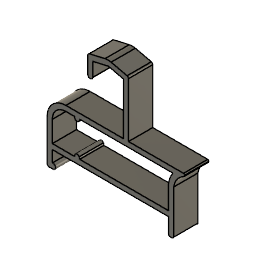
AdaptadorRiel (Autodesk Fusion 360 design; units mm, degrees)
part number: 2025-12-28-18-35-44-628
Autodesk Fusion 360 part; units mm, degrees
sketch "Boceto1" plane through (0, 0, 0) normal (0, 1, 0) x (1, 0, 0)
  line L0 (52.1, -0.6) -> (52.1, -18.5)
  line L1 (0, -17.65) -> (0, -0.6)
  line L2 (2.15, 0) -> (2.7296, 0)
  line L3 (49.95, -0.6) -> (49.95, -6.85)
  line L4 (49.95, -6.85) -> (2.15, -6.85)
  line L5 (2.15, -6.85) -> (2.15, -2.1)
  arc A0 (2.15, -2.1) -> (2.7296, 0) centre (2.4398, -1.05) ccw
  line L6 (0.6, 0) -> (2.7296, 0)
  line L7 (50.55, 0) -> (51.5, 0)
  arc A1 (0.6, 0) -> (0, -0.6) centre (0.6, -0.6) ccw
  arc A2 (50.55, 0) -> (49.95, -0.6) centre (50.55, -0.6) ccw
  arc A3 (52.1, -0.6) -> (51.5, 0) centre (51.5, -0.6) ccw
  arc A4 (0, -17.65) -> (7.75, -25.4) centre (7.75, -17.65) ccw
  line L8 (52.1, -25.4) -> (56.15, -25.4)
  line L9 (56.6, -24.95) -> (56.6, -24.7835)
  arc A5 (52.1, -18.5) -> (56.3513, -24.381) centre (59.8591, -17.3682) ccw
  arc A6 (56.15, -25.4) -> (56.6, -24.95) centre (56.15, -24.95) ccw
  arc A7 (56.6, -24.7835) -> (56.3513, -24.381) centre (56.15, -24.7835) ccw
  line L10 (2.15, -17.65) -> (2.15, -9)
  arc A8 (2.15, -17.65) -> (7.75, -23.25) centre (7.75, -17.65) ccw
  arc A9 (49.95, -18.6465) -> (51.6168, -23.0152) centre (59.8591, -17.3682) ccw
  line L11 (49.95, -9) -> (49.95, -18.6465)
  arc A10 (51.4931, -23.25) -> (51.6168, -23.0152) centre (51.4931, -23.1) ccw
  arc A11 (11.3, -9) -> (11.4993, -9.8229) centre (13.208, -8.9734) ccw
  line L12 (11.4993, -9.8229) -> (13.208, -9.8229) construction
  arc A12 (13.208, -9.8229) -> (13.4, -9) centre (11.5634, -9.0053) ccw
  arc A13 (11.4993, -9.8229) -> (13.208, -9.8229) centre (12.3537, -9.3982) ccw
  line L13 (49.95, -9) -> (13.4, -9)
  line L14 (11.3, -9) -> (2.15, -9)
  arc A14 (11.6218, -22.29) -> (11.3, -23.25) centre (12.6842, -23.18) ccw
  arc A15 (13.4, -23.25) -> (13.0782, -22.29) centre (12.0158, -23.18) ccw
  arc A16 (13.0782, -22.29) -> (11.6218, -22.29) centre (12.35, -22.9) ccw
  line L15 (51.4931, -23.25) -> (13.4, -23.25)
  line L16 (11.3, -23.25) -> (7.75, -23.25)
  line L17 (31.4, -25.4) -> (31.4, -46.6)
  line L18 (31.4, -46.6) -> (25.2, -48.1)
  line L19 (25.2, -48.1) -> (18.8, -46.6231)
  line L20 (18.8, -46.6231) -> (18.8, -40.9)
  line L21 (17.8, -39.9) -> (17.7, -39.9)
  line L22 (16.7, -40.9) -> (16.7, -47.8649)
  arc A17 (18.8, -40.9) -> (17.8, -39.9) centre (17.8, -40.9) ccw
  arc A18 (17.7, -39.9) -> (16.7, -40.9) centre (17.7, -40.9) ccw
  line L23 (23.8484, -50.1112) -> (17.2814, -48.5957)
  line L24 (26.3501, -50.1046) -> (32.9225, -48.5513)
  line L25 (33.5, -47.8214) -> (33.5, -25.4)
  line L26 (52.1, -25.4) -> (33.5, -25.4)
  line L27 (31.4, -25.4) -> (7.75, -25.4)
  arc A19 (16.7, -47.8649) -> (17.2814, -48.5957) centre (17.45, -47.8649) ccw
  arc A20 (32.9225, -48.5513) -> (33.5, -47.8214) centre (32.75, -47.8214) ccw
  arc A21 (23.8484, -50.1112) -> (26.3501, -50.1046) centre (25.0851, -44.752) ccw
  dimension "d1" = 0.6
  dimension "d2" = 7.75
  dimension "d3" = 0.45
  dimension "d5" = 0.15
  dimension "d6" = 1
  dimension "d7" = 0.75
  dimension "d8" = 5.5
  constraint horizontal L6
  constraint vertical L0
  constraint horizontal L26
  constraint vertical L1
  constraint horizontal L2
  constraint vertical L3
  constraint horizontal L4
  constraint vertical L5
  constraint coincident L2.start L6
  constraint collinear L6 L7
  constraint tangent L1 A1
  constraint tangent L6 A1
  constraint tangent L3 A2
  constraint tangent L7 A2
  constraint equal A1 A2
  constraint tangent L0 A3
  constraint tangent L7 A3
  constraint equal A1 A3
  constraint tangent A4 L26
  constraint tangent L1 A4
  constraint perpendicular L0 L8
  constraint perpendicular L8 L9
  constraint tangent L8 A6
  constraint tangent L9 A6
  constraint tangent L9 A7
  constraint tangent A5 A7
  constraint equal A6 A7
  constraint concentric A4 A8
  constraint concentric A5 A9
  constraint tangent L10 A8
  constraint tangent A8 L15
  constraint tangent A10 L15
  constraint tangent A9 A10
  constraint tangent A11 A13
  constraint coincident A11.start L13
  constraint horizontal L12
  constraint collinear L13 L14
  constraint tangent A14 A16
  constraint coincident A14.end L15
  constraint tangent A15 A16
  constraint collinear L15 L16
  constraint coincident L17.start L26
  constraint perpendicular L17 L26
  constraint vertical L20
  constraint perpendicular L20 L21
  constraint perpendicular L21 L22
  constraint tangent L20 A17
  constraint tangent L21 A17
  constraint tangent L21 A18
  constraint tangent L22 A18
  constraint equal A17 A18
  constraint parallel L19 L23
  constraint perpendicular L25 L26
  constraint collinear L26 L27
  constraint tangent L23 A19
  constraint tangent L22 A19
  constraint tangent L24 A20
  constraint tangent L25 A20
  constraint equal A19 A20
  constraint tangent L23 A21
  constraint tangent L24 A21
  measures "d1" radius of A1
  measures "d2" radius of A4
  measures "d3" radius of A6
  measures "d5" radius of A10
  measures "d6" radius of A17
  measures "d7" radius of A19
  measures "d8" radius of A21
extrude "Extruir1" add sketch "Boceto1" along normal blind 10
equation "L = 10 mm"
equation "d10 = L"
